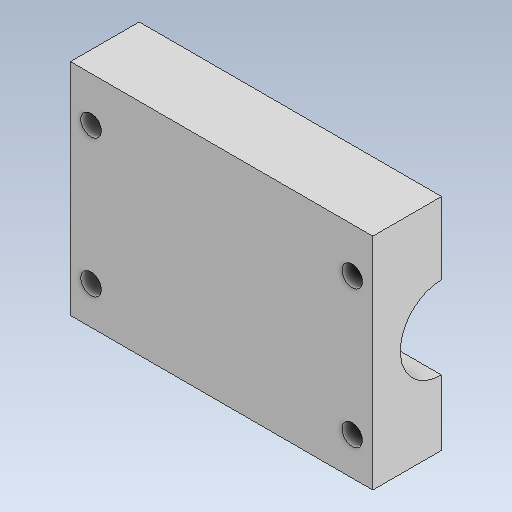
# Autodesk Inventor part: YClampTop
Saved by Autodesk Inventor 2020 (Build 240168000, 168)
## iProperties
Created: 2020-03-18
Part Number: YClampTop
Material: Generic
Document SubType Name: Modeling
Designer: DasNick
Density: 1 g/cm^3
Appearance: Default
Author: DasNick
Autodesk Inventor part; units mm, degrees
ref_plane "YZ Plane" through (0, 0, 0) normal (1, 0, 0) x (0, 1, 0)
ref_plane "XZ Plane" through (0, 0, 0) normal (0, 1, 0) x (-1, 0, 0)
ref_plane "XY Plane" through (0, 0, 0) normal (0, 0, 1) x (1, 0, 0)
sketch "Sketch1" plane through (0, 0, 0) normal (0, 0, 1) x (1, 0, 0)
  circle A0 centre (29.8858, 59.5313) radius 2.3813 projected
  circle A1 centre (-30.4392, 59.5313) radius 2.3812 projected
  circle A2 centre (-30.4392, 91.2813) radius 2.3813 projected
  circle A3 centre (29.8858, 91.2813) radius 2.3813 projected
  circle A4 centre (-30.4392, 91.2813) radius 2.3813 projected
  circle A5 centre (29.8858, 91.2813) radius 2.3813 projected
  line L0 (-35.2017, 84.9313) -> (34.6483, 84.9313) projected
  line L1 (34.6483, 84.9313) -> (34.6483, 101.6) projected
  line L2 (34.6483, 101.6) -> (-35.2017, 101.6) projected
  line L3 (-35.2017, 101.6) -> (-35.2017, 84.9313) projected
  line L4 (34.6483, 101.6) -> (-35.2017, 101.6)
  line L5 (-35.2017, 101.6) -> (-35.2017, 50.8)
  line L6 (-35.2017, 50.8) -> (34.6483, 50.8)
  line L7 (34.6483, 50.8) -> (34.6483, 101.6)
  point P0 (0, 0)
  dimension "d0" = 50.8
  constraints: 8 end point, 2 parallel, 1 horizontal, 1 perpendicular
  measures "d0" distance of L5.end L4.end
extrude "Extrusion1" add sketch "Sketch1" along normal blind 15.875
sketch "Sketch2" plane through (-35.2017, 50.8, 0) normal (-1, 0, 0) x (0, 0, 1)
  arc A0 (0, 34.1313) -> (0, 15.0813) centre (0, 24.6063) ccw projected
  circle A1 centre (0, 24.6063) radius 9.525
  point P0 (0, -50.8)
  point P1 (0, 15.0813)
  point P2 (0, 34.1313)
  constraints: 1 centre point, 1 coincident
extrude "Extrusion2" cut sketch "Sketch2" against normal blind 76.2
body "Solid1"
